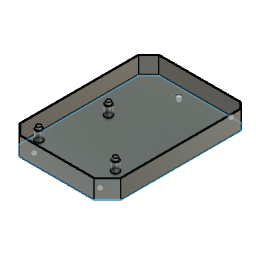
support_console_v0.1 (Autodesk Fusion 360 design; units mm, degrees)
Autodesk Fusion 360 part; units mm, degrees
sketch "Esquisse1" plane through (0, 0, 0) normal (0, 0, 1) x (1, 0, 0)
  line L0 (-67.0376, -74.6501) -> (-67.0376, 48.5999)
  line L1 (-67.0376, 48.5999) -> (-56.0775, 59.5601)
  line L2 (-67.0376, 48.5999) -> (-24.635, 48.5999) construction
  line L3 (-56.0775, 59.5601) -> (28.9225, 59.5601)
  line L4 (28.9225, 59.5601) -> (35.2865, 53.1961)
  line L5 (28.9225, 59.5601) -> (18.2996, 59.5601) construction
  line L6 (35.2865, 53.1961) -> (35.2865, -71.8039)
  line L7 (35.2865, -71.8039) -> (21.4979, -85.5925)
  line L8 (35.2865, -71.8039) -> (13.9785, -71.8039) construction
  line L9 (-67.0376, -74.6501) -> (-56.0775, -85.6102)
  line L10 (-67.0376, -74.6501) -> (-51.5916, -74.6501) construction
  line L11 (-56.0775, -85.6102) -> (21.4979, -85.5925)
  dimension "d1" = 123.25
  dimension "d3" = 15.5
  dimension "d4" = 45
  dimension "d5" = 85
  dimension "d6" = 135
  dimension "d7" = 9
  dimension "d8" = 125
  dimension "d9" = 45
  dimension "d10" = 19.5
  dimension "d11" = 45
  dimension "d12" = 15.5
  constraint vertical L0
  constraint horizontal L2
  constraint horizontal L3
  constraint horizontal L5
  constraint perpendicular L3 L6
  constraint horizontal L8
  constraint horizontal L10
  measures "d1" distance of L0.start L0.end
  measures "d3" distance of L0.end L1.end
  measures "d4" angle of L1 L2
  measures "d5" distance of L1.end L3.end
  measures "d6" angle of L4 L5
  measures "d7" distance of L3.end L4.end
  measures "d8" distance of L4.end L6.end
  measures "d9" angle of L7 L8
  measures "d10" distance of L6.end L7.end
  measures "d11" angle of L9 L10
  measures "d12" distance of L0.start L9.end
extrude "Extrusion4" add sketch "Esquisse1" along normal blind 2
extrude "Extrusion5" add sketch "Esquisse1" along normal blind 2
extrude "Extrusion6" add 1 faces at (1.1785, 9.9974, 2) along direction (0, 0, 1) blind 8 thin wall 1 inside
sketch "Esquisse6" plane through (0, 0, 2) normal (0, 0, 1) x (-1, 0, 0)
  line L0 (66.0376, -48.1857) -> (66.0376, 74.2359)
  line L1 (66.0376, 74.2359) -> (55.6633, 84.6101)
  line L2 (55.6633, 84.6101) -> (-21.0836, 84.5926)
  line L3 (-21.0836, 84.5926) -> (-34.2865, 71.3897)
  line L4 (-34.2865, 71.3897) -> (-34.2865, -52.7819)
  line L5 (-34.2865, -52.7819) -> (-28.5083, -58.5601)
  line L6 (-28.5083, -58.5601) -> (55.6632, -58.5601)
  line L7 (55.6632, -58.5601) -> (66.0376, -48.1857)
  circle A0 centre (58.6376, 62.6108) radius 3.5
  circle A1 centre (-8.7865, 50.5954) radius 3.5
  circle A2 centre (45.0376, 4.1077) radius 3.5
  dimension "d33" = 7
  dimension "d34" = 7.4
  dimension "d35" = 22
  dimension "d36" = 7
  dimension "d37" = 7
  dimension "d38" = 25.5
  dimension "d39" = 34
  dimension "d40" = 21
  dimension "d41" = 80.5
  measures "d33" diameter of A0
  measures "d34" distance of L0 A0.centre
  measures "d35" distance of L2 A0.centre
  measures "d36" diameter of A1
  measures "d37" diameter of A2
  measures "d38" distance of L4 A1.centre
  measures "d39" distance of L2 A1.centre
  measures "d40" distance of L0 A2.centre
  measures "d41" distance of L2 A2.centre
extrude "Extrusion7" add sketch "Esquisse6" along normal blind 10 contours A2
extrude "Extrusion8" add 1 faces at (34.9532, -29.9991, 10) along direction (0, 0, 1) blind 9
extrude "Extrusion9" add sketch "Esquisse6" along normal blind 10 contours A0
extrude "Extrusion10" add sketch "Esquisse6" along normal blind 10 contours A1
sketch "Esquisse8" plane through (0, 0, 12) normal (0, 0, 1) x (-1, 0, 0)
  circle A0 centre (45.0376, 4.1077) radius 3.5
  circle A1 centre (45.0376, 4.1077) radius 2.25
  dimension "d50" = 4.5
  constraint concentric A0 A1
  measures "d50" diameter of A1
extrude "Extrusion11" add sketch "Esquisse8" along normal blind 3 contours A1
sketch "Esquisse9" plane through (0, 0, 12) normal (0, 0, 1) x (-1, 0, 0)
  circle A0 centre (-8.7865, 50.5954) radius 3.5
  circle A1 centre (-8.7865, 50.5954) radius 2.25
  dimension "d53" = 4.5
  constraint concentric A0 A1
  measures "d53" diameter of A1
sketch "Esquisse10" plane through (0, 0, 12) normal (0, 0, 1) x (-1, 0, 0)
  circle A0 centre (58.6376, 62.6108) radius 3.5
  circle A1 centre (58.6376, 62.6108) radius 2.25
  dimension "d54" = 4.5
  constraint concentric A0 A1
  measures "d54" diameter of A1
extrude "Extrusion12" add sketch "Esquisse10" along normal blind 3 contours A1
extrude "Extrusion13" add sketch "Esquisse9" along normal blind 3 contours A1
extrude "Extrusion1" [suppressed]
extrude "Extrusion2" [suppressed]
extrude "Extrusion3" [suppressed]
other "SurfaceDeleteFace1"
